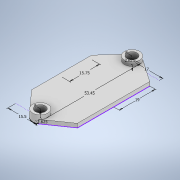
# Autodesk Inventor part: front trunk table
Saved by Autodesk Inventor 2020 (Build 240168000, 168)
## iProperties
Created: 2021-05-18
Part Number: front trunk table
Material: Generic
Document SubType Name: Modeling
Designer: Steven
Density: 1 g/cm^3
Appearance: Default
Author: Steven
Autodesk Inventor part; units mm, degrees
ref_plane "YZ Plane" through (0, 0, 0) normal (1, 0, 0) x (0, 1, 0)
ref_plane "XZ Plane" through (0, 0, 0) normal (0, 1, 0) x (-1, 0, 0)
ref_plane "XY Plane" through (0, 0, 0) normal (0, 0, 1) x (1, 0, 0)
sketch "Sketch1" plane through (0, 0, 0) normal (0, 1, 0) x (-1, 0, 0)
  line L0 (0, 0) -> (0, -53.45) construction
  line L1 (0, -53.45) -> (0, -50.825) construction
  line L2 (0, 0) -> (0, -2.625) construction
  circle A0 centre (0, -2.625) radius 2.625
  circle A1 centre (0, -50.825) radius 2.625
  circle A2 centre (0, -2.625) radius 4
  circle A3 centre (0, -50.825) radius 4
  line L3 (-2.625, -2.625) -> (12.875, -2.625) construction
  line L4 (0, -26.725) -> (12.875, -26.725) construction
  line L5 (12.875, -26.725) -> (12.875, -42.475)
  line L6 (12.875, -26.725) -> (12.875, -10.975)
  line L7 (12.875, -10.975) -> (2.9761, 0.0477)
  line L8 (12.875, -42.475) -> (2.9761, -53.4977)
  line L9 (2.625, -50.825) -> (-14.375, -50.825) construction
  line L10 (0, -26.725) -> (-14.375, -26.725) construction
  line L11 (-14.375, -26.725) -> (-14.375, -45.725)
  line L12 (-14.375, -26.725) -> (-14.375, -7.725)
  line L13 (-14.375, -7.725) -> (-2.2792, 0.6621)
  line L14 (-14.375, -45.725) -> (-2.2792, -54.1121)
  dimension "d0" = 53.45
  dimension "d1" = 2.625
  dimension "d2" = 2.625
  dimension "d3" = 8
  dimension "d4" = 8
  dimension "d5" = 15.5
  dimension "d6" = 15.75
  dimension "d7" = 17
  dimension "d8" = 19
  constraints: 30 end point, 8 point on circle, 4 centre point, 4 coincident, 4 horizontal, 4 tangent, 3 vertical, 2 point on line, 2 symmetric about line, 1 midpoint
  measures "d0" distance of L0.start L0.end
  measures "d1" distance of L0.end L1.end
  measures "d2" distance of L0.start L2.end
  measures "d3" diameter of A2
  measures "d4" diameter of A3
  measures "d5" distance of L3.start L3.end
  measures "d6" distance of L4.end L5.end
  measures "d7" distance of L9.start L9.end
  measures "d8" distance of L10.end L11.end
extrude "Extrusion1" add sketch "Sketch1" along normal blind 2 contours A2 L7 L6 L5 L8 A3 L14 L11 L12 L13
extrude "Extrusion2" add sketch "Sketch1" along normal blind 4 contours A2 | A3
body "Solid1"
